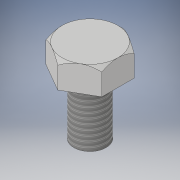
# Autodesk Inventor part: Bolt
Saved by Autodesk Inventor 2019 (Build 230136000, 136)
## iProperties
Created: 2019-05-15
Part Number: Bolt
Material: Generic
Document SubType Name: Modeling
Designer: Gustavo Marin
Density: 1 g/cm^3
Appearance: Default
Author: Gustavo Marin
Autodesk Inventor part; units mm, degrees
ref_plane "YZ Plane" through (0, 0, 0) normal (1, 0, 0) x (0, 1, 0)
ref_plane "XZ Plane" through (0, 0, 0) normal (0, 1, 0) x (-1, 0, 0)
ref_plane "XY Plane" through (0, 0, 0) normal (0, 0, 1) x (1, 0, 0)
sketch "Sketch1" plane through (0, 0, 0) normal (0, 1, 0) x (-1, 0, 0)
  line L0 (10.9985, -6.35) -> (0, -12.7)
  line L1 (0, -12.7) -> (-10.9985, -6.35)
  line L2 (-10.9985, -6.35) -> (-10.9985, 6.35)
  line L3 (-10.9985, 6.35) -> (0, 12.7)
  line L4 (0, 12.7) -> (10.9985, 6.35)
  line L5 (10.9985, 6.35) -> (10.9985, -6.35)
  point P0 (0, 0)
  point P1 (0, 0)
  dimension "d0" = 25.4
  constraints: 12 end point, 1 coincident, 1 vertical, 13 other
  measures "d0" distance of L3.end L0.end
extrude "Extrusion1" add sketch "Sketch1" along normal blind 10.16
sketch "Sketch2" plane through (0, 10.16, 0) normal (0, 1, 0) x (1, 0, 0)
  circle A0 centre (0, 0) radius 10.9985
  constraints: 1 centre point, 1 coincident
extrude "Extrusion2" cut sketch "Sketch2" against normal through all draft 45 keep common part
sketch "Sketch3" plane through (0, 0, 0) normal (0, -1, 0) x (1, 0, 0)
  circle A0 centre (0, 0) radius 6.35
  dimension "d5" = 12.7
  constraints: 1 centre point, 1 coincident
  measures "d5" diameter of A0
extrude "Extrusion3" add sketch "Sketch3" along normal blind 22.86
thread "Thread1" size "1/2-13 UNC" class "1A" standard "ANSI Unified Screw Threads" full length
body "Solid1"
